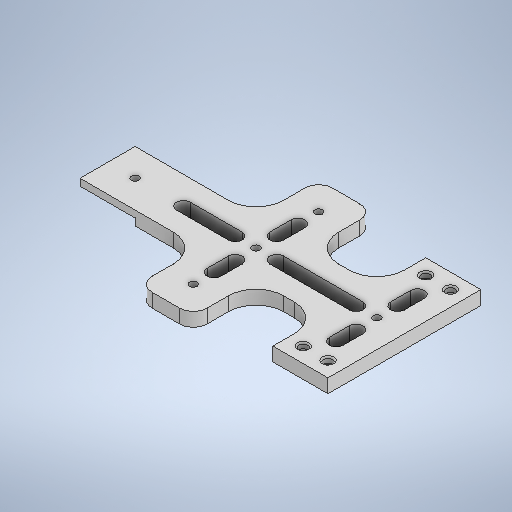
# Autodesk Inventor part: Chassis Front Spine
Saved by Autodesk Inventor 2025.2 (Build 292293000, 293)
## iProperties
Created: 2025-02-20
Part Number: Chassis Front Spine
Material: Generic
Document SubType Name: Modeling
Designer: Matt Tidd
Density: 1 g/cm^3
Appearance: Default
Author: Matt Tidd
Autodesk Inventor part; units mm, degrees
ref_plane "YZ Plane" through (0, 0, 0) normal (1, 0, 0) x (0, 1, 0)
ref_plane "XZ Plane" through (0, 0, 0) normal (0, 1, 0) x (-1, 0, 0)
ref_plane "XY Plane" through (0, 0, 0) normal (0, 0, 1) x (1, 0, 0)
sketch "Sketch1" plane through (0, 0, 0) normal (0, 1, 0) x (-1, 0, 0)
  line L0 (-20, 55.5) -> (20, 55.5)
  line L1 (20, 55.5) -> (20, -55.5)
  line L2 (20, -55.5) -> (-20, -55.5)
  line L3 (-20, -55.5) -> (-20, 55.5)
  line L4 (0, 55.5) -> (0, -55.5) construction
  line L5 (20, 0) -> (-20, 0) construction
  circle A0 centre (9, -44.5) radius 1.8
  circle A1 centre (9, 44.5) radius 1.8
  circle A2 centre (-9, -44.5) radius 1.8
  circle A3 centre (-9, 44.5) radius 1.8
  circle A4 centre (0, 0) radius 2.75
  line L6 (155.5, -20) -> (20, -20)
  line L7 (20, -20) -> (20, 20)
  line L8 (20, 20) -> (155.5, 20)
  line L9 (155.5, 20) -> (155.5, -20)
  point P0 (145, 0)
  point P1 (145, -20)
  dimension "d0" = 40
  dimension "d1" = 111
  dimension "d2" = 3.6
  dimension "d3" = 5.5
  dimension "d4" = 40
  constraints: 20 end point, 5 centre point, 5 midpoint, 4 parallel, 3 symmetric about line, 2 horizontal, 2 perpendicular, 2 point on line, 1 coincident, 3 other
  measures "d0" distance of L1.end L2.end
  measures "d1" distance of L0.end L1.end
  measures "d2" diameter of A0
  measures "d3" diameter of A4
  measures "d4" distance of L6.end L7.end
extrude "Extrusion1" add sketch "Sketch1" along normal blind 10
sketch "Sketch2" plane through (0, 10, 0) normal (0, 1, 0) x (1, 0, 0)
  circle A0 centre (-9, 44.5) radius 1.8 projected
  circle A1 centre (-9, 44.5) radius 3.25
  circle A2 centre (9, 44.5) radius 1.8 projected
  circle A3 centre (9, 44.5) radius 3.25
  circle A4 centre (9, -44.5) radius 1.8 projected
  circle A5 centre (9, -44.5) radius 3.25
  circle A6 centre (-9, -44.5) radius 1.8 projected
  circle A7 centre (-9, -44.5) radius 3.25
  point P0 (0, 0)
  dimension "d7" = 6.5
  dimension "d8" = 6.5
  dimension "d9" = 6.5
  dimension "d10" = 6.5
  constraints: 4 centre point, 4 coincident
  measures "d7" diameter of A1
  measures "d8" diameter of A3
  measures "d9" diameter of A5
  measures "d10" diameter of A7
extrude "Extrusion2" cut sketch "Sketch2" against normal blind 4
fillet "Fillet1" radius 1 4 edges at (-12.25, 10, 44.5) (5.75, 10, 44.5) (5.75, 10, -44.5) (-12.25, 10, -44.5)
fillet "Fillet2" radius 20 2 edges at (-20, 5, 20) (-20, 5, -20)
sketch "Sketch3" plane through (-155.5, 0, 20) normal (0, 0, 1) x (1, 0, 0)
  line L0 (0, 0) -> (0, 10) projected
  line L1 (0, 10) -> (-25, 10)
  line L2 (-25, 10) -> (-25, 5)
  line L3 (-25, 5) -> (0, 5)
  line L4 (0, 5) -> (0, 10)
  line L5 (0, 5) -> (15, 5)
  line L6 (15, 5) -> (15, 0)
  line L7 (15, 0) -> (0, 0)
  line L8 (0, 0) -> (0, 5)
  point P0 (155.5, 0)
  dimension "d15" = 25
  dimension "d16" = 5
  dimension "d17" = 15
  dimension "d18" = 5
  constraints: 16 end point, 4 parallel, 2 horizontal, 2 perpendicular
  measures "d15" distance of L3.end L2.end
  measures "d16" distance of L2.end L1.end
  measures "d17" distance of L6.end L7.end
  measures "d18" distance of L5.end L6.end
extrude "Extrusion3" add sketch "Sketch3" against normal blind 40 contours L3 L2 L1 L0
extrude "Extrusion4" cut sketch "Sketch3" against normal blind 40 contours L0 L5 L6 L7
sketch "Sketch4" plane through (0, 10, 0) normal (0, 1, 0) x (1, 0, 0)
  circle A0 centre (0, 0) radius 2.75 construction
  circle A1 centre (-9, 44.5) radius 1.8 construction
  circle A2 centre (9, 44.5) radius 1.8 construction
  line L0 (-9, 44.5) -> (9, 44.5) construction
  line L1 (0, 29.5) -> (0, 15) construction
  line L2 (-5, 29.5) -> (-5, 15)
  line L3 (5, 15) -> (5, 29.5)
  arc A3 (5, 29.5) -> (-5, 29.5) centre (0, 29.5) ccw
  arc A4 (-5, 15) -> (5, 15) centre (0, 15) ccw
  line L4 (-7.5, 0) -> (7.5, 0) construction
  line L5 (-5, -29.5) -> (-5, -15)
  line L6 (5, -15) -> (5, -29.5)
  arc A5 (-5, -29.5) -> (5, -29.5) centre (0, -29.5) ccw
  arc A6 (5, -15) -> (-5, -15) centre (0, -15) ccw
  line L7 (-160.5, 0) -> (0, 0) construction
  line L8 (-40, 20) -> (-140.5, 20) construction
  line L9 (-140.5, -20) -> (-140.5, 20) construction
  line L10 (-140.5, 20) -> (-140.5, -20) construction
  point P0 (0, 22.25)
  point P1 (-95.25, 0)
  point P2 (-65.25, 0)
  point P3 (-15, 0)
  point P4 (-125.5, 0)
  dimension "d33" = 10
  dimension "d34" = 15
  constraints: 20 end point, 8 point on circle, 6 symmetric about line, 4 centre point, 4 tangent, 3 horizontal, 3 point on line, 2 midpoint, 1 parallel, 1 vertical, 2 other
  measures "d33" diameter of A4
  measures "d34" distance of L4.start L4.end
extrude "Extrusion5" cut sketch "Sketch4" against normal blind 10
sketch "Sketch5" plane through (-40, 0, 20) normal (0, 0, 1) x (1, 0, 0)
  line L0 (0, 10) -> (-140.5, 10) projected
  line L1 (-140.5, 10) -> (-155.5, 10)
  line L2 (-155.5, 10) -> (-155.5, 5)
  line L3 (-155.5, 5) -> (-140.5, 5)
  line L4 (-140.5, 5) -> (-140.5, 10)
  line L5 (-100.5, 0) -> (-100.5, 5) projected
  line L6 (-100.5, 5) -> (-115.5, 5)
  line L7 (-115.5, 5) -> (-115.5, 0)
  line L8 (-115.5, 0) -> (-100.5, 0)
  line L9 (-100.5, 0) -> (-100.5, 5)
  point P0 (40, 0)
  dimension "d49" = 15
  dimension "d53" = 15
  dimension "d54" = 5
  constraints: 16 end point, 4 parallel, 2 horizontal, 2 perpendicular
  measures "d49" distance of L3.end L2.end
  measures "d53" distance of L8.end L7.end
  measures "d54" distance of L7.end L6.end
extrude "Extrusion6" add sketch "Sketch5" against normal blind 40
sketch "Sketch6" plane through (0, 10, 0) normal (0, 1, 0) x (1, 0, 0)
  circle A0 centre (-175.5, 0) radius 2.75
  line L0 (-175.5, 0) -> (0, 0) construction
  circle A1 centre (-87.75, 0) radius 2.75
  line L1 (-155.5, -20) -> (-155.5, 20) construction
  line L2 (-155.5, -20) -> (-155.5, 20) construction
  line L3 (-140.5, 0) -> (-102.75, 0) construction
  line L4 (-140.5, -5) -> (-102.75, -5)
  line L5 (-102.75, 5) -> (-140.5, 5)
  arc A2 (-140.5, 5) -> (-140.5, -5) centre (-140.5, 0) ccw
  arc A3 (-102.75, -5) -> (-102.75, 5) centre (-102.75, 0) ccw
  line L6 (-72.75, 0) -> (-15, 0) construction
  line L7 (-72.75, -5) -> (-15, -5)
  line L8 (-15, 5) -> (-72.75, 5)
  arc A4 (-72.75, 5) -> (-72.75, -5) centre (-72.75, 0) ccw
  arc A5 (-15, -5) -> (-15, 5) centre (-15, 0) ccw
  point P0 (-155.5, 0)
  point P1 (-121.625, 0)
  point P2 (-43.875, 0)
  dimension "d55" = 5.5
  dimension "d58" = 87.75
  dimension "d63" = 10
  dimension "d64" = 10
  constraints: 20 end point, 8 point on circle, 8 tangent, 6 centre point, 4 midpoint, 4 point on line, 3 collinear, 2 horizontal, 2 parallel, 2 other
  measures "d55" diameter of A0
  measures "d58" distance of L0.start A1.centre
  measures "d63" diameter of A3
  measures "d64" diameter of A5
extrude "Extrusion7" cut sketch "Sketch6" against normal through all
sketch "Sketch8" plane through (0, 10, 0) normal (0, 1, 0) x (1, 0, 0)
  circle A0 centre (-87.75, 0) radius 2.75 projected
  line L0 (-87.75, -20) -> (-87.75, 20) construction
  line L1 (-40, 20) -> (-155.5, 20) projected
  line L2 (-107.75, 20) -> (-67.75, 20) construction
  line L3 (-107.75, -20) -> (-67.75, -20) construction
  line L4 (-155.5, -20) -> (-40, -20) construction
  line L5 (-107.75, 20) -> (-67.75, 20)
  line L6 (-67.75, 20) -> (-67.75, 65.5)
  line L7 (-67.75, 65.5) -> (-107.75, 65.5)
  line L8 (-107.75, 65.5) -> (-107.75, 20)
  line L9 (-107.75, -20) -> (-67.75, -20)
  line L10 (-67.75, -20) -> (-67.75, -65.5)
  line L11 (-67.75, -65.5) -> (-107.75, -65.5)
  line L12 (-107.75, -65.5) -> (-107.75, -20)
  point P0 (0, 0)
  dimension "d67" = 40
  dimension "d68" = 40
  dimension "d69" = 45.5
  dimension "d70" = 45.5
  constraints: 22 end point, 4 parallel, 4 point on line, 3 midpoint, 2 horizontal, 2 perpendicular, 1 vertical
  measures "d67" distance of L2.start L2.end
  measures "d68" distance of L3.start L3.end
  measures "d69" distance of L6.end L5.end
  measures "d70" distance of L9.end L10.end
extrude "Extrusion8" add sketch "Sketch8" against normal blind 10 contours L1 L8 L7 L6 | L9 L10 L11 L12
sketch "Sketch9" plane through (0, 10, 0) normal (0, 1, 0) x (1, 0, 0)
  circle A0 centre (-87.75, 0) radius 2.75 construction
  line L0 (20, 0) -> (-195.5, 0) construction
  line L1 (-195.5, -20) -> (-195.5, 20) construction
  line L2 (-87.75, -65.5) -> (-87.75, 65.5) construction
  line L3 (-107.75, 65.5) -> (-67.75, 65.5) construction
  circle A1 centre (-87.75, -45.5) radius 2.75
  circle A2 centre (-87.75, 45.5) radius 2.75
  line L4 (-87.75, -30.5) -> (-87.75, -15) construction
  line L5 (-82.75, -30.5) -> (-82.75, -15)
  line L6 (-92.75, -15) -> (-92.75, -30.5)
  arc A3 (-92.75, -30.5) -> (-82.75, -30.5) centre (-87.75, -30.5) ccw
  arc A4 (-82.75, -15) -> (-92.75, -15) centre (-87.75, -15) ccw
  line L7 (-87.75, 15) -> (-87.75, 30.5) construction
  line L8 (-82.75, 15) -> (-82.75, 30.5)
  line L9 (-92.75, 30.5) -> (-92.75, 15)
  arc A5 (-92.75, 15) -> (-82.75, 15) centre (-87.75, 15) ccw
  arc A6 (-82.75, 30.5) -> (-92.75, 30.5) centre (-87.75, 30.5) ccw
  point P0 (0, 0)
  point P1 (-87.75, -22.75)
  point P2 (-87.75, 22.75)
  dimension "d74" = 5.5
  dimension "d75" = 10
  dimension "d76" = 10
  constraints: 20 end point, 8 point on circle, 8 tangent, 6 centre point, 6 midpoint, 5 point on line, 2 collinear, 2 parallel, 1 symmetric about line, 1 other
  measures "d74" diameter of A1
  measures "d75" diameter of A4
  measures "d76" diameter of A6
extrude "Extrusion9" cut sketch "Sketch9" against normal blind 10
fillet "Fillet4" radius 20 4 edges at (-67.75, 5, 20) (-67.75, 5, -20) (-107.75, 5, -20) (-107.75, 5, 20)
fillet "Fillet5" radius 10 4 edges at (-67.75, 5, 65.5) (-107.75, 5, 65.5) (-107.75, 5, -65.5) (-67.75, 5, -65.5)
body "Solid1"
